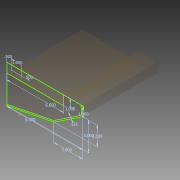
# Autodesk Inventor part: ramp1
Saved by Autodesk Inventor 2011 SP1 (Build 150282100, 282)
## iProperties
Created: 2012-01-19
Part Number: ramp1
Document SubType Name: Modeling
Designer: Christopher
Density: 1 g/cm^3
Author: Christopher
Autodesk Inventor part; units mm, degrees
ref_plane "YZ Plane" through (0, 0, 0) normal (1, 0, 0) x (0, 1, 0)
ref_plane "XZ Plane" through (0, 0, 0) normal (0, 1, 0) x (-1, 0, 0)
ref_plane "XY Plane" through (0, 0, 0) normal (0, 0, 1) x (1, 0, 0)
sketch "Sketch1" plane through (0, 0, 0) normal (0, 0, 1) x (1, 0, 0)
  line L0 (169.4484, 80.0625) -> (169.4484, 105.4625)
  line L1 (169.4484, 105.4625) -> (166.2734, 105.4625)
  line L2 (-33.7516, 3.8625) -> (-33.7516, 105.4625)
  line L3 (-33.7516, 105.4625) -> (166.2734, 105.4625)
  line L4 (-33.7516, 105.4625) -> (118.6484, 105.4625)
  line L5 (118.6484, 105.4625) -> (118.6484, 80.0625)
  line L6 (118.6484, 80.0625) -> (-33.7516, 80.0625)
  line L7 (-33.7516, 80.0625) -> (-33.7516, 105.4625)
  line L8 (169.4484, 80.0625) -> (93.2484, 29.2625)
  line L9 (93.2484, 29.2625) -> (-33.7516, 3.8625)
  line L10 (92.0098, 32.2527) -> (166.2734, 81.7618)
  line L11 (166.2734, 102.2875) -> (166.2734, 102.2875)
  line L12 (166.2734, 81.7618) -> (166.2734, 105.4625)
  line L13 (-33.7516, 7.1687) -> (92.1562, 32.3503)
  line L14 (118.6484, 105.4625) -> (166.2734, 105.4625)
  line L15 (-33.7516, 7.1687) -> (-33.7516, 80.0625)
  point P0 (0, 0)
  point P1 (-21.0516, 92.7625)
  point P2 (4.3484, 92.7625)
  dimension "d2" = 25.4
  dimension "d3" = 203.2
  dimension "d4" = 76.2
  dimension "d15" = 12.7
  dimension "d16" = 25.4
  dimension "d17" = 12.7
  dimension "d25" = 152.4
  dimension "d26" = 25.4
  dimension "d29" = 50.8
  dimension "d30" = 76.2
  dimension "d31" = 3.175
  constraints: 32 end point, 4 parallel, 3 perpendicular, 2 collinear, 2 point on line, 1 horizontal, 1 horizontal alignment, 1 vertical
  measures "d2" distance of L0.start L0.end
  measures "d3" distance from line of L2.start L0
  measures "d4" vertical distance of L2.start L0.start
  measures "d15" distance from line of L2 point (-21.052, 92.763)
  measures "d16" distance of point (4.348, 92.763) point (-21.052, 92.763)
  measures "d17" distance from line of L3 point (-21.052, 92.763)
  measures "d25" distance of L5.end L6.end
  measures "d26" distance of L4.end L5.end
  measures "d29" vertical distance of L0.start L8.end
  measures "d30" distance from line of L0 L8.end
  measures "d31" distance between parallel lines of L8 L10
extrude "Extrusion1" add sketch "Sketch1" against normal blind 203.2 contours L8 L9 L2 L13 L10 L12 L1 L0
extrude "Extrusion3" add sketch "Sketch1" against normal blind 3.175
sketch "Sketch2" plane through (0, 0, -203.2) normal (0, 0, -1) x (-1, 0, 0)
  line L0 (-169.4484, 80.0625) -> (-169.4484, 105.4625) projected
  line L1 (33.7516, 3.8625) -> (-169.4484, 80.0625) projected
  line L2 (-169.4484, 105.4625) -> (-166.2734, 105.4625) projected
  line L3 (-166.2734, 105.4625) -> (33.7516, 105.4625)
  line L4 (33.7516, 105.4625) -> (33.7516, 3.8625)
  line L5 (-93.2484, 29.2625) -> (-169.4484, 80.0625) projected
  line L6 (33.7516, 3.8625) -> (-93.2484, 29.2625) projected
  line L7 (-166.2734, 81.7618) -> (-166.2734, 105.4625) projected
  line L8 (-93.2484, 29.2625) -> (-169.4484, 80.0625)
  line L9 (-169.4484, 80.0625) -> (-169.4484, 105.4625)
  line L10 (-169.4484, 105.4625) -> (-166.2734, 105.4625)
  line L11 (-166.2734, 105.4625) -> (-166.2734, 81.7618)
  line L12 (-92.1562, 32.3503) -> (-166.2734, 81.7618)
  line L13 (33.7516, 3.8625) -> (-93.2484, 29.2625)
  line L14 (-92.1562, 32.3503) -> (33.7516, 7.1687)
  point P0 (0, 0)
  constraints: 18 end point, 6 collinear, 2 parallel, 1 perpendicular
extrude "Extrusion4" add sketch "Sketch2" against normal blind 3.175
hole "Hole1" at (-21.0516, 92.7625, 0) at (4.3484, 92.7625, 0) direction (0, 0, -1) diameter 6.35 depth 254 tip angle 118
extrude "Extrusion5" cut sketch "Sketch1" against normal blind 228.6 contours L5 L6 L2 L3
body "Solid1"
